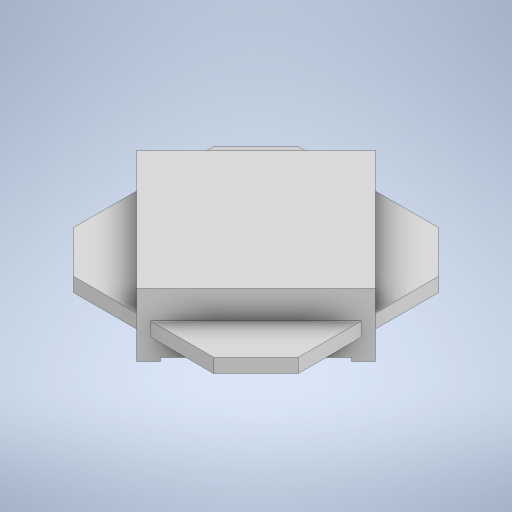
# Autodesk Inventor part: Liyue_Vision_Base
Saved by Autodesk Inventor 2024 (Build 280153000, 153)
## iProperties
Created: 2024-08-26
Part Number: Liyue_Vision_Base
Material: Generic
Document SubType Name: Modeling
Designer: Malik
Density: 1 g/cm^3
Appearance: Default
Author: Malik
Autodesk Inventor part; units mm, degrees
ref_plane "YZ Plane" through (0, 0, 0) normal (1, 0, 0) x (0, 1, 0)
ref_plane "XZ Plane" through (0, 0, 0) normal (0, 1, 0) x (-1, 0, 0)
ref_plane "XY Plane" through (0, 0, 0) normal (0, 0, 1) x (1, 0, 0)
sketch "Sketch1" plane through (0, 0, 0) normal (0, 1, 0) x (-1, 0, 0)
  line L0 (0, 0) -> (-101.6, 0)
  line L1 (-101.6, 0) -> (-101.6, -101.6)
  line L2 (-101.6, -101.6) -> (0, -101.6)
  line L3 (0, -101.6) -> (0, 0)
  dimension "d0" = 101.6
  dimension "d1" = 101.6
  constraints: 8 end point, 2 parallel, 1 horizontal, 1 perpendicular
  measures "d0" distance of L2.end L1.end
  measures "d1" distance of L1.end L0.end
extrude "Extrusion1" add sketch "Sketch1" along normal mid plane 6.35
chamfer "Chamfer1" distance 19.05 angle 45 4 edges at (101.6, 0, -101.6) (101.6, 0, 0) (0, 0, 0) (0, 0, -101.6)
sketch "Sketch2" plane through (0, 3.175, 0) normal (0, 1, 0) x (1, 0, 0)
  line L0 (101.6, 19.05) -> (101.6, 82.55) projected
  line L1 (0, 82.55) -> (0, 19.05) projected
  line L2 (19.05, 0) -> (82.55, 0) projected
  line L3 (82.55, 101.6) -> (19.05, 101.6) projected
  line L4 (50.8, 101.6) -> (0, 50.8)
  line L5 (50.8, 0) -> (0, 50.8)
  line L6 (50.8, 0) -> (101.6, 50.8)
  line L7 (101.6, 50.8) -> (50.8, 101.6)
  line L8 (104.775, 50.8) -> (50.8, 104.775)
  line L9 (50.8, 104.775) -> (-3.175, 50.8)
  line L10 (-3.175, 50.8) -> (50.8, -3.175)
  line L11 (50.8, -3.175) -> (104.775, 50.8)
  point P0 (0, 0)
  point P1 (50.8, 50.8)
  point P2 (-3.175, 50.8)
  dimension "d8" = 3.175
  dimension "d9" = 3.175
  dimension "d10" = 3.175
  constraints: 16 end point, 6 midpoint, 6 perpendicular
  measures "d8" distance of point (0, 50.8) point (-3.175, 50.8)
  measures "d9" distance of point (50.8, 0) L10.end
  measures "d10" distance of L8.end L4.start
extrude "Extrusion2" add sketch "Sketch2" along normal mid plane 25.4
sketch "Sketch3" plane through (0, -9.525, 0) normal (0, -1, 0) x (1, 0, 0)
  line L0 (104.775, -50.8) -> (99.3868, -45.4118)
  line L1 (101.6, -47.625) -> (53.975, 0) projected
  line L2 (99.3868, -45.4118) -> (93.9987, -50.8)
  line L3 (93.9987, -50.8) -> (99.3868, -56.1882)
  line L4 (53.975, -101.6) -> (101.6, -53.975) projected
  line L5 (99.3868, -56.1882) -> (104.775, -50.8)
  line L6 (-3.175, -50.8) -> (50.8, -104.775) construction
  line L7 (99.3868, -45.4118) -> (104.775, -50.8) construction
  line L8 (99.3868, -45.4118) -> (104.775, -50.8) construction
  line L9 (-3.175, -50.8) -> (2.2132, -45.4118)
  line L10 (2.2132, -45.4118) -> (7.6013, -50.8)
  line L11 (7.6013, -50.8) -> (2.2132, -56.1882)
  line L12 (2.2132, -56.1882) -> (-3.175, -50.8)
  line L13 (-3.175, -50.8) -> (50.8, 3.175) construction
  line L14 (50.8, -104.775) -> (45.4118, -99.3868)
  line L15 (45.4118, -99.3868) -> (50.8, -93.9987)
  line L16 (50.8, -93.9987) -> (56.1882, -99.3868)
  line L17 (56.1882, -99.3868) -> (50.8, -104.775)
  line L18 (50.8, 3.175) -> (56.1882, -2.2132)
  line L19 (56.1882, -2.2132) -> (50.8, -7.6013)
  line L20 (50.8, -7.6013) -> (45.4118, -2.2132)
  line L21 (45.4118, -2.2132) -> (50.8, 3.175)
  line L22 (77.7875, -77.7875) -> (23.8125, -23.8125) construction
  line L23 (56.1882, -2.2132) -> (99.3868, -45.4118) construction
  line L24 (53.4941, -4.9072) -> (96.6928, -48.1059)
  line L25 (51.5687, -6.8326) -> (94.7674, -50.0313)
  line L26 (97.4818, -47.3168) -> (54.2832, -4.1182)
  line L27 (47.625, -101.6) -> (0, -53.975)
  line L28 (4.9072, -53.4941) -> (48.1059, -96.6928)
  line L29 (6.8326, -51.5687) -> (50.0313, -94.7674)
  line L30 (47.3168, -97.4818) -> (4.1182, -54.2832)
  line L31 (94.7607, -51.562) -> (51.562, -94.7607)
  line L32 (97.4818, -54.2832) -> (54.2832, -97.4818)
  line L33 (56.1882, -99.3868) -> (99.3868, -56.1882)
  line L34 (96.6944, -53.4958) -> (53.4958, -96.6944)
  line L35 (77.7875, -23.8125) -> (23.8125, -77.7875) construction
  line L36 (0, -47.625) -> (47.625, 0)
  line L37 (50.038, -6.8393) -> (6.8393, -50.038)
  line L38 (47.3168, -4.1182) -> (4.1182, -47.3168)
  line L39 (48.1042, -4.9056) -> (4.9056, -48.1042)
  point P0 (0, 0)
  point P1 (4.1182, -54.2832)
  dimension "d16" = 1.905
  dimension "d19" = 1.905
  dimension "d20" = 0.762
  dimension "d21" = 0.7874
  constraints: 73 end point, 16 symmetric about line, 12 point on line, 9 perpendicular, 6 midpoint, 4 collinear
  measures "d16" horizontal distance of L26.start L0.end
  measures "d19" horizontal distance of L32.start L3.end
  measures "d20" horizontal distance of L31.start L2.end
  measures "d21" horizontal distance of L34.start L32.start
extrude "Extrusion3" add sketch "Sketch3" along normal blind 3.175 contours L5 L4 L3 L2 L0 | L19 L20 L21 L18 L1 | L4 L17 L14 L15 L16 | L10 L11 L12 L9
extrude "Extrusion4" add sketch "Sketch3" along normal blind 1.5875 contours L2 L26 L19 L1 | L4 L16 L32 L3 | L2 L25 L19 L24 | L34 L16 L31 L3 | L20 L38 L10 L36 | L27 L11 L30 L15 | L37 L10 L39 L20 | L15 L28 L11 L29
body "Solid1"
